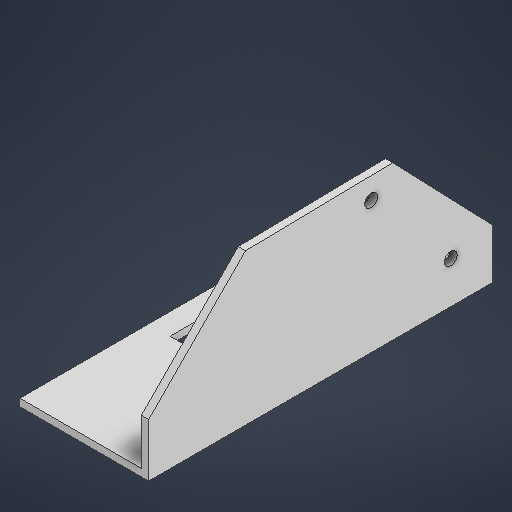
# Autodesk Inventor part: gripper servo mount
Saved by Autodesk Inventor 2026 (Build 300175050, 175E)
## iProperties
Created: 2025-05-22
Part Number: gripper servo mount
Material: Generic
Document SubType Name: Modeling
Designer: Verchasv
Density: 1 g/cm^3
Appearance: Default
Author: Verchasv
Autodesk Inventor part; units mm, degrees
ref_plane "YZ Plane" through (0, 0, 0) normal (1, 0, 0) x (0, 1, 0)
ref_plane "XZ Plane" through (0, 0, 0) normal (0, 1, 0) x (-1, 0, 0)
ref_plane "XY Plane" through (0, 0, 0) normal (0, 0, 1) x (1, 0, 0)
sketch "Sketch1" plane through (0, 0, 0) normal (0, 1, 0) x (-1, 0, 0)
  line L0 (0, 0) -> (20, 0)
  line L1 (20, 0) -> (20, -40)
  line L2 (20, -40) -> (0, -40)
  line L3 (0, -40) -> (0, 0)
  line L4 (25, 30) -> (-5, 30)
  line L5 (-5, 30) -> (-5, -50)
  line L6 (-5, -50) -> (25, -50)
  line L7 (25, -50) -> (25, 30)
  dimension "d0" = 20
  dimension "d1" = 40
  dimension "d2" = 30
  dimension "d3" = 30
  dimension "d4" = 10
  dimension "d5" = 5
  constraints: 16 end point, 4 parallel, 2 horizontal, 2 perpendicular
  measures "d0" distance of L1.end L2.end
  measures "d1" distance of L0.end L1.end
  measures "d2" distance of L4.start L4.end
  measures "d3" distance between parallel lines of L0 L4
  measures "d4" distance between parallel lines of L2 L6
  measures "d5" distance between parallel lines of L5 L3
extrude "Extrusion1" add sketch "Sketch1" along normal blind 1.7
sketch "Sketch2" plane through (5, 0, 30) normal (1, 0, 0) x (0, 0, -1)
  line L0 (0, 0) -> (0, 1.7) projected
  line L1 (0, 1.7) -> (0, 12.4073)
  line L2 (0, 12.4073) -> (22.5503, 35.1708)
  line L3 (22.5503, 35.1708) -> (56.8462, 35.7913)
  line L4 (56.8462, 35.7913) -> (80, 11.7)
  line L5 (80, 0) -> (80, 1.7) projected
  line L6 (80, 11.7) -> (80, 1.7)
  line L7 (0, 1.7) -> (80, 1.7) projected
  circle A0 centre (70.3665, 9.7) radius 1.5
  circle A1 centre (70.3665, 9.7) radius 28
  line L8 (24.8863, 30.7) -> (59.3173, 30.7)
  circle A2 centre (51.8462, 30.7) radius 1.5
  point P0 (30, 0)
  dimension "d11" = 56
  dimension "d8" = 0
  dimension "d9" = 3
  dimension "d10" = 8
  dimension "d12" = 29
  dimension "d13" = 3
  dimension "d14" = 5
  dimension "d15" = 5
  dimension "d16" = 10
  constraints: 12 end point, 2 centre point, 1 coincident, 1 horizontal, 1 point on line, 1 vertical, 3 other
  measures "d8" horizontal distance of L5.end L4.end
  measures "d9" diameter of A0
  measures "d10" distance from line of L7 A0.centre
  measures "d12" distance between parallel lines of L7 L8
  measures "d13" diameter of A2
  measures "d14" horizontal distance of L3.end A2.centre
  measures "d15" distance from line of L3 A2.centre
  measures "d16" distance of L4.end L5.end
extrude "Extrusion2" add sketch "Sketch2" against normal blind 1.7 contours L1 L2 L3 L4 A1 A2 L7 | A1 A2 L4 L6 L7
sketch "Sketch5" plane through (0, 0, 0) normal (0, -1, 0) x (1, 0, 0)
  circle A0 centre (-5.663, -44.592) radius 1.5
  circle A1 centre (-13.663, -44.592) radius 1.5
  line L0 (-25, -50) -> (-25, 30) projected
  line L1 (5, -50) -> (-25, -50) projected
  point P0 (0, 0)
  dimension "d21" = 3
  dimension "d22" = 3
  dimension "d23" = 8
  dimension "d24" = 11.337
  dimension "d27" = 5.408
  dimension "d28" = 5.408
  constraints: 2 centre point
  measures "d21" diameter of A0
  measures "d22" diameter of A1
  measures "d23" distance of A1.centre A0.centre
  measures "d24" distance from line of L0 A1.centre
  measures "d27" distance from line of L1 A1.centre
  measures "d28" distance from line of L1 A0.centre
extrude "Extrusion3" cut sketch "Sketch5" against normal blind 10
body "Solid1"
